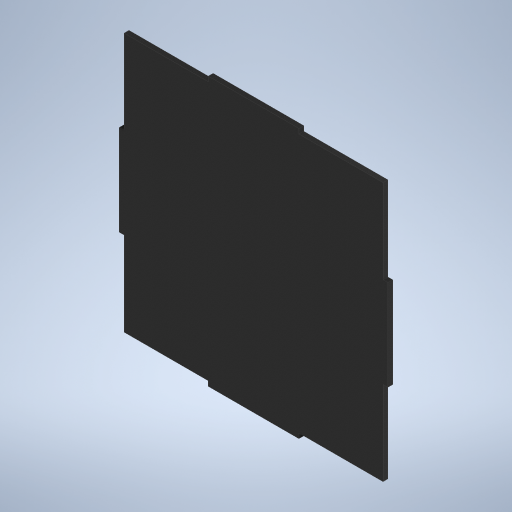
# Autodesk Inventor part: Final Product backplate
Saved by Autodesk Inventor 2024.2 (Build 282272000, 272)
## iProperties
Created: 2024-02-22
Part Number: Final Product backplate
Material: Generic
Document SubType Name: Modeling
Designer: flynf
Density: 1 g/cm^3
Appearance: Black Cast
Author: flynf
Autodesk Inventor part; units mm, degrees
ref_plane "YZ Plane" through (0, 0, 0) normal (1, 0, 0) x (0, 1, 0)
ref_plane "XZ Plane" through (0, 0, 0) normal (0, 1, 0) x (-1, 0, 0)
ref_plane "XY Plane" through (0, 0, 0) normal (0, 0, 1) x (1, 0, 0)
sketch "Sketch1" plane through (0, 0, 0) normal (0, 0, 1) x (1, 0, 0)
  line L0 (0, 0) -> (-1016, 0)
  line L1 (-1016, 0) -> (-1016, 1016)
  line L2 (-1016, 1016) -> (0, 1016)
  line L3 (0, 1016) -> (0, 0)
  line L4 (19.05, 1035.05) -> (-1035.05, 1035.05)
  line L5 (-1035.05, 1035.05) -> (-1035.05, -19.05)
  line L6 (-1035.05, -19.05) -> (19.05, -19.05)
  line L7 (19.05, -19.05) -> (19.05, 1035.05)
  line L8 (-685.8, 1016) -> (-685.8, 1035.05)
  line L9 (-330.2, 1016) -> (-330.2, 1035.05)
  line L10 (-685.8, -19.05) -> (-685.8, 0)
  line L11 (-330.2, -19.05) -> (-330.2, 0)
  line L12 (0, 330.2) -> (19.05, 330.2)
  line L13 (0, 685.8) -> (19.05, 685.8)
  line L14 (-1016, 685.8) -> (-1035.05, 685.8)
  line L15 (-1016, 330.2) -> (-1035.05, 330.2)
  point P0 (-1644.65, 1016)
  point P1 (-1644.65, 1035.05)
  point P2 (-387.35, 1016)
  point P3 (-387.35, 1035.05)
  point P4 (-685.8, -19.05)
  point P5 (-685.8, 0)
  point P6 (-330.2, 0)
  point P7 (-330.2, -19.05)
  dimension "d0" = 1016
  dimension "d1" = 1016
  dimension "d2" = 19.05
  dimension "d5" = 355.6
  dimension "d7" = 355.6
  dimension "d10" = 349.25
  dimension "d11" = 349.25
  dimension "d12" = 355.6
  dimension "d13" = 349.25
  dimension "d14" = 349.25
  dimension "d15" = 349.25
  dimension "d18" = 349.25
  constraints: 32 end point, 16 point on line, 6 perpendicular, 5 parallel, 2 horizontal, 3 other
  measures "d0" distance of L1.end L2.end
  measures "d1" distance of L0.end L1.end
  measures "d2" distance between parallel lines of L2 L4
  measures "d5" distance between parallel lines of L9 L8
  measures "d7" distance between parallel lines of L11 L10
  measures "d10" distance between parallel lines of L12 L6
  measures "d11" distance between parallel lines of L4 L13
  measures "d12" distance between parallel lines of L13 L12
  measures "d13" distance between parallel lines of L5 L10
  measures "d14" distance between parallel lines of L4 L14
  measures "d15" distance between parallel lines of L6 L15
  measures "d18" distance between parallel lines of L7 L9
extrude "Extrusion1" add sketch "Sketch1" along normal blind 19.05 contours L0 L1 L2 L3 | L11 L6 L10 L0 | L3 L13 L7 L12 | L15 L5 L14 L1 | L2 L8 L4 L9
body "Solid1"
